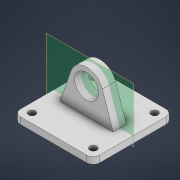
# Autodesk Inventor part: Replacement_Front_Lower Arm
Saved by Autodesk Inventor 2022 (Build 260153000, 153)
## iProperties
Created: 2024-06-22
Part Number: Replacement_Front_Lower Arm
Material: Generic
Document SubType Name: Modeling
Designer: Todd McKenzie
Density: 1 g/cm^3
Appearance: Default
Author: Todd McKenzie
Autodesk Inventor part; units mm, degrees
ref_plane "YZ Plane" through (0, 0, 0) normal (1, 0, 0) x (0, 1, 0)
ref_plane "XZ Plane" through (0, 0, 0) normal (0, 1, 0) x (-1, 0, 0)
ref_plane "XY Plane" through (0, 0, 0) normal (0, 0, 1) x (1, 0, 0)
sketch "Sketch1" plane through (0, 0, 0) normal (0, 1, 0) x (-1, 0, 0)
  point P0 (0, 0)
sketch "Sketch2" plane through (0, 0, 0) normal (0, 1, 0) x (-1, 0, 0)
  line L0 (5.5728, 34.4065) -> (41.025, 34.4065)
  arc A0 (47.375, 28.0565) -> (41.025, 34.4065) centre (41.025, 28.0565) ccw
  line L1 (47.375, 28.0565) -> (47.375, -0.9482)
  line L2 (47.375, -0.9482) -> (47.375, -35.4435)
  arc A1 (41.025, -41.7935) -> (47.375, -35.4435) centre (41.025, -35.4435) ccw
  line L3 (41.025, -41.7935) -> (3.9588, -41.7935)
  line L4 (5.5728, 34.4065) -> (-22.475, 34.4065)
  line L5 (-28.825, 28.0565) -> (-28.825, -35.4435)
  line L6 (3.9588, -41.7935) -> (-22.475, -41.7935)
  arc A2 (-28.825, -35.4435) -> (-22.475, -41.7935) centre (-22.475, -35.4435) ccw
  arc A3 (-22.475, 34.4065) -> (-28.825, 28.0565) centre (-22.475, 28.0565) ccw
  circle A4 centre (38.6374, 25.6689) radius 3.3782
  circle A5 centre (38.6374, -33.0559) radius 3.3782
  circle A6 centre (-20.0874, 25.6689) radius 3.3782
  circle A7 centre (-20.0874, -33.0559) radius 3.3782
  point P0 (0, 0)
  point P1 (47.375, -0.9482)
  dimension "d0" = 76.2
  dimension "d1" = 76.2
  dimension "d2" = 6.7564
  dimension "d3" = 8.7376
  dimension "d4" = 8.7376
  dimension "d5" = 6.7564
  dimension "d6" = 8.7376
  dimension "d7" = 8.7376
  dimension "d8" = 6.7564
  dimension "d9" = 8.7376
  dimension "d10" = 8.7376
  dimension "d11" = 6.7564
  dimension "d12" = 8.7376
  dimension "d13" = 8.7376
  dimension "d42" = 6.35
  constraints: 14 end point, 8 centre point, 8 point on circle, 8 tangent, 4 horizontal, 3 equal radius, 3 vertical, 1 coincident
  measures "d0" distance between parallel lines of L5 L1
  measures "d1" distance between parallel lines of L3 L0
  measures "d2" diameter of A4
  measures "d3" distance from line of L1 A4.centre
  measures "d4" distance from line of L0 A4.centre
  measures "d5" diameter of A5
  measures "d6" distance from line of L2 A5.centre
  measures "d7" distance from line of A5.centre L3
  measures "d8" diameter of A6
  measures "d9" distance from line of A6.centre L5
  measures "d10" distance from line of A6.centre L4
  measures "d11" diameter of A7
  measures "d12" distance from line of A7.centre L5
  measures "d13" distance from line of L6 A7.centre
  measures "d42" radius of A1
extrude "Extrusion1" add sketch "Sketch2" along normal blind 6.35
sketch "Sketch4" plane through (-41.025, 0, 34.4065) normal (0, 0, 1) x (1, 0, 0)
  line L0 (0, 6.35) -> (63.5, 6.35) projected
  line L1 (6.35, 6.35) -> (16.7195, 36.8587)
  line L2 (6.35, 6.35) -> (57.15, 6.35)
  line L3 (57.15, 6.35) -> (46.7805, 36.8587)
  line L4 (-6.35, 0) -> (-6.35, 6.35) projected
  line L5 (69.85, 0) -> (69.85, 6.35) projected
  line L6 (7.5688, 6.35) -> (57.15, 6.35)
  arc A0 (46.7805, 36.8587) -> (16.7195, 36.8587) centre (31.75, 31.75) ccw
  line L7 (7.5688, 6.35) -> (57.15, 6.35)
  circle A1 centre (31.75, 31.75) radius 11.4808
  point P0 (41.025, 0)
  dimension "d18" = 15.875
  dimension "d21" = 22.9616
  dimension "d23" = 25.4
  dimension "d24" = 25.4
  dimension "d25" = 12.7
  dimension "d27" = 25.4
  constraints: 10 end point, 2 centre point, 2 point on circle, 2 point on line, 2 tangent, 1 coincident, 1 collinear, 1 horizontal
  measures "d18" radius of A0
  measures "d21" diameter of A1
  measures "d23" horizontal distance of L1.start A0.centre
  measures "d24" horizontal distance of L2.end A0.centre
  measures "d25" distance from line of L5 L2.end
  measures "d27" distance from line of L0 A0.centre
extrude "Extrusion2" add sketch "Sketch4" against normal blind 76.2
sketch "Sketch5" plane through (-47.375, 0, -35.4435) normal (-1, 0, 0) x (0, 0, 1)
  line L0 (-6.35, 6.35) -> (25.4, 6.35)
  line L1 (25.4, 6.35) -> (25.4, 47.625)
  line L2 (-6.35, 47.625) -> (-6.35, 36.8587) projected
  line L3 (25.4, 47.625) -> (-6.35, 47.625)
  line L4 (-6.35, 6.35) -> (-6.35, 36.8587) projected
  line L5 (-6.35, 47.625) -> (-6.35, 6.35)
  point P0 (35.4435, 0)
  dimension "d30" = 31.75
  dimension "d31" = 90
  constraints: 8 end point, 1 horizontal
  measures "d30" distance of L0.start L0.end
  measures "d31" angle of L0 L1
extrude "Extrusion3" cut sketch "Sketch5" against normal blind 76.2
ref_plane "Work Plane2" through (22.475, 0, -3.6935) normal (0, 0, -1) x (-1, 0, 0)
mirror "Mirror1" about plane through (22.475, 0, -3.6935) normal (0, 0, -1) of "Extrusion3"
body "Solid1"
